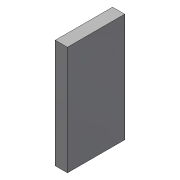
# Autodesk Inventor part: BLANK-BC-10004
Saved by Autodesk Inventor 2016 (Build 200138000, 138)
## iProperties
Created: 2015-12-02
Part Number: BLANK-BC-10004
Project: DIPOLO BC-3T- SIRIUS
Cost Center: 1504002005
Material: Aço Carbono
Document SubType Name: Modeling
Designer: reinaldo.basilio
Density: 7.87 g/cm^3
Appearance: Steel
Mass: 20898.5 g
Surface Area: 1685.74 cm^2
Volume: 2655.47 cm^3
Description: Base do polo do dipolo de baixo campo.
RuleStatus: InUse
AfterMaterialChange0: file://_iMaterial
AfterAnyiPropertyChange0: file://_iMaterial
AfterDocNew0: file://_Naming_par
AfterDocNew1: file://_NameStart
AfterDocNew2: file://_NameStart1
AfterDocNew3: file://_Materiais
DocNumber: XXXXX-XXX-XXXX-00-001.ipt
Folder: .
Title: DIPOLO BC-3T- SIRIUS
Author: reinaldo.basilio
Subject: BLANK-BC-10004
Autodesk Inventor part; units mm, degrees
ref_plane "YZ Plane" through (0, 0, 0) normal (1, 0, 0) x (0, 1, 0)
ref_plane "XZ Plane" through (0, 0, 0) normal (0, 1, 0) x (-1, 0, 0)
ref_plane "XY Plane" through (0, 0, 0) normal (0, 0, 1) x (1, 0, 0)
sketch "Sketch5" plane through (0, 0, 0) normal (0, 1, 0) x (-1, 0, 0)
  line L0 (89.5, -170) -> (89.5, 170)
  line L1 (-89.5, 170) -> (89.5, 170)
  line L2 (-89.5, -170) -> (-89.5, 170)
  line L3 (89.5, -170) -> (-89.5, -170)
  point P0 (0, 0)
  point P1 (0, 0)
  point P2 (70, 0)
  dimension "d8" = 340
  dimension "d9" = 179
  dimension "d26" = 89.5
  dimension "d27" = 170
  constraints: 8 end point, 2 horizontal, 2 vertical
  measures "d8" distance of L2.start L1.start
  measures "d9" distance of L1.start L0.end
  measures "d26" distance from line of L0 point (0, 0)
  measures "d27" distance from line of L1 point (0, 0)
extrude "Extrusion5" add sketch "Sketch5" along normal mid plane 38
equation "\"d26\" = 0.5 * d9"
equation "\"d27\" = 0.5 * d8"
body "Solid5"
